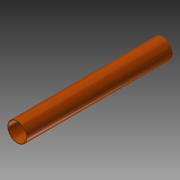
# Autodesk Inventor part: Liner
Saved by Autodesk Inventor 2015 (Build 190159000, 159)
## iProperties
Created: 2016-01-09
Part Number: Liner
Material: Phenolic Resin
Document SubType Name: Modeling
Designer: Jared
Density: 1.38 g/cm^3
Appearance: Smooth - Light Orange
Author: Jared
Autodesk Inventor part; units mm, degrees
ref_plane "YZ Plane" through (0, 0, 0) normal (1, 0, 0) x (0, 1, 0)
ref_plane "XZ Plane" through (0, 0, 0) normal (0, 1, 0) x (-1, 0, 0)
ref_plane "XY Plane" through (0, 0, 0) normal (0, 0, 1) x (1, 0, 0)
sketch "Sketch1" plane through (0, 0, 0) normal (0, 0, 1) x (1, 0, 0)
  circle A0 centre (0, 0) radius 71.4375
  circle A1 centre (0, 0) radius 65.8876
  dimension "d0" = 142.875
  dimension "d1" = 131.7752
  constraints: 2 centre point, 2 coincident
  measures "d0" diameter of A0
  measures "d1" diameter of A1
extrude "Extrusion1" add sketch "Sketch1" along normal blind 1050.925
body "Solid1"
